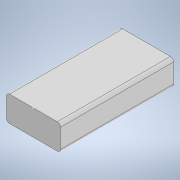
# Autodesk Inventor part: PX9200-23A_LIPO_Battery
Saved by Autodesk Inventor 2022.3 (Build 263350000, 350)
## iProperties
Created: 2022-07-07
Part Number: PX9200-23A_LIPO_Battery
Material: Generic
Document SubType Name: Modeling
Designer: luis_
Density: 1 g/cm^3
Appearance: Default
Author: luis_
Autodesk Inventor part; units mm, degrees
ref_plane "YZ Plane" through (0, 0, 0) normal (1, 0, 0) x (0, 1, 0)
ref_plane "XZ Plane" through (0, 0, 0) normal (0, 1, 0) x (-1, 0, 0)
ref_plane "XY Plane" through (0, 0, 0) normal (0, 0, 1) x (1, 0, 0)
sketch "Sketch3" plane through (0, 0, 0) normal (0, 0, 1) x (1, 0, 0)
  line L0 (-17, -8) -> (17, -8)
  line L1 (17, -8) -> (17, 8)
  line L2 (17, 8) -> (-17, 8)
  line L3 (-17, 8) -> (-17, -8)
  line L4 (-17, -8) -> (17, 8) construction
  line L5 (17, -8) -> (-17, 8) construction
  point P0 (0, 0)
  dimension "d4" = 34
  dimension "d5" = 16
  constraints: 12 end point, 2 midpoint, 2 parallel, 1 horizontal, 1 perpendicular
  measures "d4" distance of L2.end L1.end
  measures "d5" distance of L1.end L0.end
extrude "Extrusion2" add sketch "Sketch3" against normal blind 71
sketch "Sketch4" plane through (-17, 8, 0) normal (0, 1, 0) x (1, 0, 0)
  point P0 (17, 0)
fillet "Fillet1" radius 2 4 edges at (17, 8, -35.5) (-17, 8, -35.5) (-17, -8, -35.5) (17, -8, -35.5)
body "Solid1"
